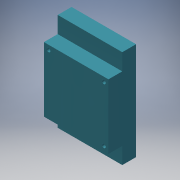
# Autodesk Inventor part: actuator
Saved by Autodesk Inventor 2018 (Build 220112000, 112)
## iProperties
Created: 2018-08-29
Part Number: actuator
Material: Generic
Document SubType Name: Modeling
Designer: David
Density: 1 g/cm^3
Appearance: Cadet Blue
Author: David
Autodesk Inventor part; units mm, degrees
ref_plane "YZ Plane" through (0, 0, 0) normal (1, 0, 0) x (0, 1, 0)
ref_plane "XZ Plane" through (0, 0, 0) normal (0, 1, 0) x (-1, 0, 0)
ref_plane "XY Plane" through (0, 0, 0) normal (0, 0, 1) x (1, 0, 0)
sketch "Sketch1" plane through (0, 0, 0) normal (0, 1, 0) x (-1, 0, 0)
  line L0 (-17.5, -17.5) -> (17.5, -17.5)
  line L1 (17.5, -17.5) -> (17.5, 17.5)
  line L2 (17.5, 17.5) -> (-17.5, 17.5)
  line L3 (-17.5, 17.5) -> (-17.5, -17.5)
  line L4 (-17.5, -17.5) -> (17.5, 17.5) construction
  line L5 (17.5, -17.5) -> (-17.5, 17.5) construction
  point P0 (0, 0)
  dimension "d0" = 35
  dimension "d1" = 35
  constraints: 12 end point, 2 midpoint, 2 parallel, 1 horizontal, 1 perpendicular
  measures "d0" distance of L2.end L1.end
  measures "d1" distance of L1.end L0.end
extrude "Extrusion1" add sketch "Sketch1" along normal blind 15
sketch "Sketch2" plane through (0, 15, 0) normal (0, 1, 0) x (1, 0, 0)
  circle A0 centre (15, -15) radius 1
  circle A1 centre (-15, -15) radius 1
  circle A2 centre (15, 15) radius 1
  point P0 (0, 0)
  dimension "d10" = 2
  dimension "d11" = 15
  dimension "d12" = 15
  dimension "d13" = 2
  dimension "d14" = 15
  dimension "d15" = 15
  dimension "d16" = 2
  dimension "d17" = 15
  dimension "d18" = 15
  constraints: 3 centre point
  measures "d10" diameter of A0
  measures "d11" horizontal distance of point (0, 0) A0.centre
  measures "d12" horizontal distance of point (0, 0) A0.centre
  measures "d13" diameter of A1
  measures "d14" horizontal distance of point (0, 0) A1.centre
  measures "d15" horizontal distance of point (0, 0) A1.centre
  measures "d16" diameter of A2
  measures "d17" horizontal distance of point (0, 0) A2.centre
  measures "d18" horizontal distance of point (0, 0) A2.centre
extrude "Extrusion2" cut sketch "Sketch2" against normal blind 15
sketch "Sketch3" plane through (17.5, 0, -17.5) normal (0, 0, -1) x (-1, 0, 0)
  line L0 (0, 0) -> (0, 15) projected
  line L1 (35, 0) -> (35, 15) projected
  line L2 (0, 15) -> (35, 15)
  line L3 (35, 15) -> (35, 7.5)
  line L4 (35, 7.5) -> (0, 7.5)
  line L5 (0, 7.5) -> (0, 15)
  point P0 (17.5, 0)
  constraints: 8 end point, 2 parallel, 1 horizontal, 1 midpoint, 1 perpendicular
extrude "Extrusion3" add sketch "Sketch3" along normal blind 9
sketch "Sketch4" plane through (-17.5, 0, 17.5) normal (0, 0, 1) x (1, 0, 0)
  line L0 (0, 15) -> (35, 15) projected
  line L1 (0, 7.5) -> (35, 7.5) projected
  line L2 (0, 15) -> (35, 15)
  line L3 (35, 15) -> (35, 7.5)
  line L4 (35, 7.5) -> (0, 7.5)
  line L5 (0, 7.5) -> (0, 15)
  point P0 (17.5, 0)
  constraints: 8 end point, 2 parallel, 1 horizontal, 1 perpendicular
extrude "Extrusion4" add sketch "Sketch4" along normal blind 9
sketch "Sketch5" plane through (0, 15, 0) normal (0, 1, 0) x (1, 0, 0)
  circle A0 centre (4.5, -15.5) radius 1.25
  line L0 (-17.5, -26.5) -> (-17.5, 26.5) projected
  line L1 (-17.5, 0) -> (17.5, 0)
  line L2 (17.5, 26.5) -> (17.5, -26.5) projected
  line L3 (0, -26.5) -> (0, 26.5)
  line L4 (-26.5, 0) -> (8.5, 0)
  circle A1 centre (-4.5, -15.5) radius 1.25
  line L5 (-17.5, 31) -> (17.5, 31)
  circle A2 centre (4.5, 15.5) radius 1.25
  line L6 (-26.5, 31) -> (8.5, 31)
  circle A3 centre (-4.5, 15.5) radius 1.25
  point P0 (0, 0)
  dimension "d25" = 15.5
  dimension "d26" = 4.5
  dimension "d27" = 2.5
  dimension "d30" = 9
  dimension "d33" = 31
  constraints: 10 end point, 4 centre point, 2 midpoint, 2 vertical, 1 collinear, 1 horizontal, 14 other
  measures "d25" vertical distance of point (0, 0) A0.centre
  measures "d26" horizontal distance of point (0, 0) A0.centre
  measures "d27" diameter of A0
  measures "d30" distance of L1.start L4.start
  measures "d33" distance of L1.start L5.start
extrude "Extrusion5" cut sketch "Sketch5" against normal blind 2
body "Solid1"
